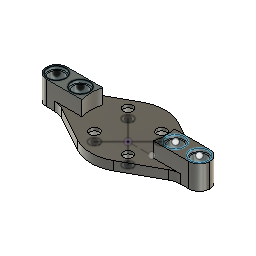
Motor_mount (Autodesk Fusion 360 design; units mm, degrees)
Autodesk Fusion 360 part; units mm, degrees
sketch "Sketch2" plane through (0, 0, 0) normal (0, 0, 1) x (1, 0, 0)
  line L0 (-21.3111, -3.5) -> (-24.01, -3.5)
  line L1 (-27.5, -0.01) -> (-27.5, 0.01)
  line L2 (-24.01, 3.5) -> (-21.3111, 3.5)
  line L3 (27.5, 0.01) -> (27.5, -0.01)
  arc A0 (-27.5, -0.01) -> (-24.01, -3.5) centre (-24.01, -0.01) ccw
  arc A1 (-24.01, 3.5) -> (-27.5, 0.01) centre (-24.01, 0.01) ccw
  arc A2 (27.5, 0.01) -> (24.01, 3.5) centre (24.01, 0.01) ccw
  arc A3 (24.01, -3.5) -> (27.5, -0.01) centre (24.01, -0.01) ccw
  circle A4 centre (24, 0) radius 2.5
  circle A5 centre (-24, 0) radius 2.5
  circle A6 centre (6.7175, 6.7175) radius 1.65
  circle A7 centre (-5.6569, 5.6569) radius 1.65
  circle A8 centre (-6.7175, -6.7175) radius 1.65
  circle A9 centre (5.6569, -5.6569) radius 1.65
  circle A10 centre (0, 0) radius 12.5
  line L4 (-17.9244, 4.3738) -> (-6.0478, 10.9396)
  line L5 (-17.9244, -4.3738) -> (-6.0478, -10.9396)
  line L6 (17.9244, 4.3738) -> (6.0478, 10.9396)
  line L7 (17.9244, -4.3738) -> (6.0478, -10.9396)
  arc A11 (-21.3111, 3.5) -> (-17.9244, 4.3738) centre (-21.3111, 10.5) ccw
  arc A12 (-17.9244, -4.3738) -> (-21.3111, -3.5) centre (-21.3111, -10.5) ccw
  line L8 (24.01, 3.5) -> (21.3111, 3.5)
  line L9 (24.01, -3.5) -> (21.3111, -3.5)
  arc A13 (21.3111, -3.5) -> (17.9244, -4.3738) centre (21.3111, -10.5) ccw
  arc A14 (17.9244, 4.3738) -> (21.3111, 3.5) centre (21.3111, 10.5) ccw
  line L10 (21.3111, -3.5) -> (12, -3.5)
  line L11 (-12, -3.5) -> (-21.3111, -3.5)
  line L12 (-21.3111, 3.5) -> (-12, 3.5)
  line L13 (12, 3.5) -> (21.3111, 3.5)
  line L14 (-16.3799, 2.0847) -> (-27.5, 3.5) construction
  line L15 (-27.5, -3.5) -> (-16.3799, -2.0847) construction
  line L16 (-12.4, -1.5782) -> (12.4, 1.5782) construction
  line L17 (25.3613, 3.2278) -> (27.5, 3.5) construction
  line L18 (27.5, -3.5) -> (25.3613, -3.2278) construction
  line L19 (12.4, -1.5782) -> (-12.4, 1.5782) construction
  circle A15 centre (-16.01, 0.01) radius 2.5
  circle A16 centre (16, 0) radius 2.5
  dimension "d42" = 9.5
  dimension "d44" = 8
  dimension "d45" = 8
  dimension "d46" = 9.5
  dimension "d47" = 55
  dimension "d48" = 7
  dimension "d49" = 3.49
  dimension "d50" = 3.49
  dimension "d51" = 3.49
  dimension "d52" = 3.49
  dimension "d53" = 24
  dimension "d54" = 5
  dimension "d55" = 24
  dimension "d56" = 5
  dimension "d61" = 3.3
  dimension "d62" = 3.3
  dimension "d63" = 3.3
  dimension "d64" = 3.3
  dimension "d65" = 25
  dimension "d66" = 7
  dimension "d67" = 7
  dimension "d68" = 7
  dimension "d69" = 7
  dimension "d92" = 8
  dimension "d93" = 8
  dimension "d94" = 5
  dimension "d95" = 5
  constraint horizontal L0
  constraint perpendicular L0 L1
  constraint parallel L0 L2
  constraint parallel L1 L3
  constraint coincident A10.centre L18
  constraint coincident A10.centre L15
  constraint coincident L15.start L1
  constraint coincident L15.start L0
  constraint tangent L1 A0
  constraint tangent L0 A0
  constraint coincident L14.end L1
  constraint coincident L14.end L2
  constraint tangent L1 A1
  constraint tangent L2 A1
  constraint coincident L17.end L2
  constraint coincident L17.end L3
  constraint tangent L2 A2
  constraint tangent L3 A2
  constraint coincident L18.start L0
  constraint coincident L18.start L3
  constraint tangent L0 A3
  constraint tangent L3 A3
  constraint coincident A10.centre origin
  constraint coincident A10 L4.end
  constraint tangent A10 L4
  constraint coincident A10 L5.end
  constraint tangent A10 L5
  constraint coincident A10 L6.end
  constraint tangent A10 L6
  constraint coincident A10 L7.end
  constraint tangent A10 L7
  constraint coincident L2 A2.end
  constraint tangent L2 A11
  constraint tangent L4 A11
  constraint coincident L0 A3.start
  constraint tangent L5 A12
  constraint tangent L0 A12
  constraint tangent L7 A13
  constraint tangent L9 A13
  constraint tangent L6 A14
  constraint tangent L8 A14
  constraint tangent A14 L12
  constraint tangent A12 L10
  constraint coincident A10 L10.end
  constraint coincident A10 L11.start
  constraint collinear L10 L11
  constraint coincident A10 L12.end
  constraint coincident A10 L13.start
  constraint collinear L12 L13
  constraint coincident L14.start L18
  constraint collinear L14 L18
  constraint coincident A10 L19.end
  constraint collinear L15 L16
  constraint coincident A10 L16.start
  constraint collinear L16 L17
  constraint collinear L18 L19
  constraint coincident A3 L18.end
  constraint coincident A2 L17.start
  constraint coincident A10 L16.end
  constraint coincident A10 L19.start
  measures "d42" distance of A10.centre A6.centre
  measures "d44" distance of A10.centre A7.centre
  measures "d45" distance of A10.centre A9.centre
  measures "d46" distance of A10.centre A8.centre
  measures "d47" distance of L14.end L17.end
  measures "d48" distance of L15.start L14.end
  measures "d49" radius of A0
  measures "d50" radius of A1
  measures "d51" radius of A2
  measures "d52" radius of A3
  measures "d53" distance of A10.centre A4.centre
  measures "d54" diameter of A4
  measures "d55" distance of A10.centre A5.centre
  measures "d56" diameter of A5
  measures "d61" diameter of A6
  measures "d62" diameter of A7
  measures "d63" diameter of A8
  measures "d64" diameter of A9
  measures "d65" diameter of A10
  measures "d66" radius of A11
  measures "d67" radius of A12
  measures "d68" radius of A13
  measures "d69" radius of A14
  measures "d92" distance of A1.centre A15.centre
  measures "d93" distance of A4.centre A16.centre
  measures "d94" diameter of A15
  measures "d95" diameter of A16
extrude "Extrude1" add sketch "Sketch2" along normal blind 8 contours L0 L1 L2 A0 A1 A10 L11 L12 | A15 makes body 1
extrude "Extrude2" add sketch "Sketch2" along normal blind 8 separate body contours L3 A2 A3 A10 L8 L9 L10 L13 | A16 makes body 2
extrude "Extrude3" add sketch "Sketch2" along normal blind 3 separate body contours A10 L5 A12 L11 | A10 | A10 L4 A11 L12 | A10 L7 A13 L10 | A10 L6 A14 L13 makes body 3
sketch "Sketch3" plane through (0, 0, 0) normal (0, 0, 1) x (1, 0, 0)
  circle A0 centre (-15, 0) radius 3.1
  circle A1 centre (-24, 0) radius 3.1
  circle A2 centre (15, 0) radius 3.1
  circle A3 centre (24, 0) radius 3.1
  dimension "d76" = 6.2
  dimension "d77" = 6.2
  dimension "d78" = 6.2
  dimension "d79" = 6.2
  measures "d76" diameter of A0
  measures "d77" diameter of A1
  measures "d78" diameter of A2
  measures "d79" diameter of A3
extrude "Extrude4" cut sketch "Sketch3" along normal blind 1 contours A1 bodies 1
extrude "Extrude7" cut sketch "Sketch3" along normal blind 1 contours A3 bodies 2
chamfer "Chamfer1" distance 2 distance2 1 1 edges at (4.1185, -5.0602, 0) measured on face at (7.3048, -5.7391, 2) on bodies 3
chamfer "Chamfer2" distance 2 distance2 1 3 edges at (-8.2559, -6.1208, 0) (-7.1952, 6.2535, 0) (5.1792, 7.3142, 0) measured on face at (-5.0696, -6.7998, 2) measured on face at (-4.0089, 5.5746, 2) measured on face at (8.3655, 6.6353, 2) on bodies 3
extrude "Extrude8" cut sketch "Sketch2" along normal blind 10 contours A15 bodies 1
extrude "Extrude9" cut sketch "Sketch2" along normal blind 10 contours A16 bodies 2
sketch "Sketch4" plane through (0, 0, 0) normal (0, 0, 1) x (1, 0, 0)
  circle A0 centre (-16, 0) radius 3
  circle A1 centre (16, 0) radius 3
  dimension "d100" = 6
  dimension "d101" = 6
  measures "d100" diameter of A0
  measures "d101" diameter of A1
extrude "Extrude10" cut sketch "Sketch4" along normal blind 1 contours A0 bodies 1
extrude "Extrude11" cut sketch "Sketch4" along normal blind 1 contours A1 bodies 2
sketch "Sketch5" plane through (0, 0, 0) normal (0, 0, 1) x (1, 0, 0)
  line L0 (0, 0) -> (5.6569, 5.6569)
  line L1 (0, 0) -> (8, 0) construction
  line L2 (0, 0) -> (-5.6569, -5.6569)
  line L3 (0, 0) -> (6.7175, -6.7175)
  line L4 (0, 0) -> (-6.7175, 6.7175)
  circle A0 centre (-6.7175, 6.7175) radius 1.65
  circle A1 centre (6.7175, -6.7175) radius 1.65
  circle A2 centre (-5.6569, -5.6569) radius 1.65
  circle A3 centre (5.6569, 5.6569) radius 1.65
  dimension "d106" = 8
  dimension "d107" = 45
  dimension "d108" = 8
  dimension "d109" = 9.5
  dimension "d110" = 9.5
  dimension "d111" = 3.3
  dimension "d112" = 3.3
  dimension "d113" = 3.3
  dimension "d114" = 3.3
  constraint horizontal L1
  constraint coincident L0.start L1.start
  constraint parallel L0 L2
  constraint perpendicular L2 L3
  constraint perpendicular L0 L4
  constraint coincident L4.end A0.centre
  constraint coincident L3.end A1.centre
  constraint coincident L2.end A2.centre
  constraint coincident L0.end A3.centre
  measures "d106" distance of L0.start L0.end
  measures "d107" angle of L0 L1
  measures "d108" distance of L0.start L2.end
  measures "d109" distance of L0.start L3.end
  measures "d110" distance of L0.start L4.end
  measures "d111" diameter of A0
  measures "d112" diameter of A1
  measures "d113" diameter of A2
  measures "d114" diameter of A3
extrude "Extrude12" add sketch "Sketch2" along normal blind 3 contours A10 | A6 | A7 | A8 | A9 bodies 3 2 1
extrude "Extrude13" cut sketch "Sketch5" along normal blind 10 contours A2 bodies 3
extrude "Extrude14" cut sketch "Sketch5" along normal blind 10 contours A0 | A1 | A3 bodies 3
chamfer "Chamfer3" distance 1 distance2 2 4 edges at (-7.1952, -6.2535, 0) (5.1792, -7.3142, 0) (-8.2559, 6.1208, 0) (4.1185, 5.0602, 0) measured on face at (1.9475, -1.9853, 0) measured on face at (1.9475, -1.9853, 0) measured on face at (1.9475, -1.9853, 0) measured on face at (1.9475, -1.9853, 0) on bodies 3
sketch "Sketch6" plane through (0, 0, 8) normal (0, 0, 1) x (-1, 0, 0)
  circle A0 centre (16.01, -0.01) radius 2.5
  circle A1 centre (24, 0) radius 2.5
  arc A2 (24.01, -3.5) -> (27.5, -0.01) centre (24.01, -0.01) ccw
  line L0 (27.5, -0.01) -> (27.5, 0.01)
  arc A3 (27.5, 0.01) -> (24.01, 3.5) centre (24.01, 0.01) ccw
  line L1 (24.01, 3.5) -> (12, 3.5)
  arc A4 (12, -3.5) -> (12, 3.5) centre (0, 0) ccw
  line L2 (12, -3.5) -> (24.01, -3.5)
  circle A5 centre (-16, 0) radius 3
  circle A6 centre (-24, 0) radius 3
  circle A7 centre (16.01, -0.01) radius 3
  circle A8 centre (24.01, 0.01) radius 3
  dimension "d123" = 6
  dimension "d124" = 6
  dimension "d125" = 6
  dimension "d126" = 6
  constraint concentric A0 A7
  constraint concentric A3 A8
  measures "d123" diameter of A5
  measures "d124" diameter of A6
  measures "d125" diameter of A7
  measures "d126" diameter of A8
extrude "Extrude15" cut sketch "Sketch6" against normal blind 1 contours A6 bodies 3
extrude "Extrude16" cut sketch "Sketch6" against normal blind 1 contours A0 | A5 | A7 | A8 bodies 3
combine "Combine1" [suppressed]
